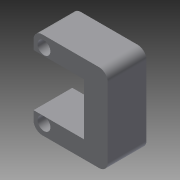
# Autodesk Inventor part: thermo-model
Saved by Autodesk Inventor 2014 (Build 180170000, 170)
## iProperties
Created: 2014-07-20
Part Number: thermo-model
Material: Generic
Document SubType Name: Modeling
Designer: james
Density: 1 g/cm^3
Appearance: Default
Author: james
Autodesk Inventor part; units mm, degrees
ref_plane "YZ Plane" through (0, 0, 0) normal (1, 0, 0) x (0, 1, 0)
ref_plane "XZ Plane" through (0, 0, 0) normal (0, 1, 0) x (-1, 0, 0)
ref_plane "XY Plane" through (0, 0, 0) normal (0, 0, 1) x (1, 0, 0)
sketch "Sketch1" plane through (0, 0, 0) normal (0, 1, 0) x (-1, 0, 0)
  spline S0 degree 3 poles (19.0088, -20.3781) (18.4587, -20.3781) (18.0142, -19.9334) (18.0142, -19.3832) (18.0142, -18.833) (18.4587, -18.3883) (19.0088, -18.3883) (19.5594, -18.3883) (20.0038, -18.833) (20.0038, -19.3832) (20.0038, -19.9334) (19.5594, -20.3781) (19.0088, -20.3781) knots 0 0 0 0 1 1 1 2 2 2 3 3 3 4 4 4 4
  line L0 (19.0088, -20.3781) -> (18.4587, -20.3781) construction
  line L1 (18.4587, -20.3781) -> (18.0142, -19.9334) construction
  line L2 (18.0142, -19.9334) -> (18.0142, -19.3832) construction
  line L3 (18.0142, -19.3832) -> (18.0142, -18.833) construction
  line L4 (18.0142, -18.833) -> (18.4587, -18.3883) construction
  line L5 (18.4587, -18.3883) -> (19.0088, -18.3883) construction
  line L6 (19.0088, -18.3883) -> (19.5594, -18.3883) construction
  line L7 (19.5594, -18.3883) -> (20.0038, -18.833) construction
  line L8 (20.0038, -18.833) -> (20.0038, -19.3832) construction
  line L9 (20.0038, -19.3832) -> (20.0038, -19.9334) construction
  line L10 (20.0038, -19.9334) -> (19.5594, -20.3781) construction
  line L11 (19.5594, -20.3781) -> (19.0088, -20.3781) construction
  spline S1 degree 3 poles (19.0088, -20.3781) (18.4587, -20.3781) (18.0142, -19.9334) (18.0142, -19.3832) (18.0142, -18.833) (18.4587, -18.3883) (19.0088, -18.3883) (19.5594, -18.3883) (20.0038, -18.833) (20.0038, -19.3832) (20.0038, -19.9334) (19.5594, -20.3781) (19.0088, -20.3781) knots 0 0 0 0 1 1 1 2 2 2 3 3 3 4 4 4 4
  line L12 (19.0088, -20.3781) -> (18.4587, -20.3781) construction
  line L13 (18.4587, -20.3781) -> (18.0142, -19.9334) construction
  line L14 (18.0142, -19.9334) -> (18.0142, -19.3832) construction
  line L15 (18.0142, -19.3832) -> (18.0142, -18.833) construction
  line L16 (18.0142, -18.833) -> (18.4587, -18.3883) construction
  line L17 (18.4587, -18.3883) -> (19.0088, -18.3883) construction
  line L18 (19.0088, -18.3883) -> (19.5594, -18.3883) construction
  line L19 (19.5594, -18.3883) -> (20.0038, -18.833) construction
  line L20 (20.0038, -18.833) -> (20.0038, -19.3832) construction
  line L21 (20.0038, -19.3832) -> (20.0038, -19.9334) construction
  line L22 (20.0038, -19.9334) -> (19.5594, -20.3781) construction
  line L23 (19.5594, -20.3781) -> (19.0088, -20.3781) construction
  spline S2 degree 3 poles (19.0088, -5.1804) (18.4587, -5.1804) (18.0142, -4.7359) (18.0142, -4.1855) (18.0142, -3.6352) (18.4587, -3.1907) (19.0088, -3.1907) (19.5594, -3.1907) (20.0038, -3.6352) (20.0038, -4.1855) (20.0038, -4.7359) (19.5594, -5.1804) (19.0088, -5.1804) knots 0 0 0 0 1 1 1 2 2 2 3 3 3 4 4 4 4
  line L24 (19.0088, -5.1804) -> (18.4587, -5.1804) construction
  line L25 (18.4587, -5.1804) -> (18.0142, -4.7359) construction
  line L26 (18.0142, -4.7359) -> (18.0142, -4.1855) construction
  line L27 (18.0142, -4.1855) -> (18.0142, -3.6352) construction
  line L28 (18.0142, -3.6352) -> (18.4587, -3.1907) construction
  line L29 (18.4587, -3.1907) -> (19.0088, -3.1907) construction
  line L30 (19.0088, -3.1907) -> (19.5594, -3.1907) construction
  line L31 (19.5594, -3.1907) -> (20.0038, -3.6352) construction
  line L32 (20.0038, -3.6352) -> (20.0038, -4.1855) construction
  line L33 (20.0038, -4.1855) -> (20.0038, -4.7359) construction
  line L34 (20.0038, -4.7359) -> (19.5594, -5.1804) construction
  line L35 (19.5594, -5.1804) -> (19.0088, -5.1804) construction
  spline S3 degree 3 poles (19.0088, -5.1804) (18.4587, -5.1804) (18.0142, -4.7359) (18.0142, -4.1855) (18.0142, -3.6352) (18.4587, -3.1907) (19.0088, -3.1907) (19.5594, -3.1907) (20.0038, -3.6352) (20.0038, -4.1855) (20.0038, -4.7359) (19.5594, -5.1804) (19.0088, -5.1804) knots 0 0 0 0 1 1 1 2 2 2 3 3 3 4 4 4 4
  line L36 (19.0088, -5.1804) -> (18.4587, -5.1804) construction
  line L37 (18.4587, -5.1804) -> (18.0142, -4.7359) construction
  line L38 (18.0142, -4.7359) -> (18.0142, -4.1855) construction
  line L39 (18.0142, -4.1855) -> (18.0142, -3.6352) construction
  line L40 (18.0142, -3.6352) -> (18.4587, -3.1907) construction
  line L41 (18.4587, -3.1907) -> (19.0088, -3.1907) construction
  line L42 (19.0088, -3.1907) -> (19.5594, -3.1907) construction
  line L43 (19.5594, -3.1907) -> (20.0038, -3.6352) construction
  line L44 (20.0038, -3.6352) -> (20.0038, -4.1855) construction
  line L45 (20.0038, -4.1855) -> (20.0038, -4.7359) construction
  line L46 (20.0038, -4.7359) -> (19.5594, -5.1804) construction
  line L47 (19.5594, -5.1804) -> (19.0088, -5.1804) construction
  line L48 (19.0302, -21.9233) -> (19.4746, -21.9019)
  spline S4 degree 3 poles (19.4746, -21.9019) (20.5647, -21.6366) (21.3157, -20.9538) (21.5279, -19.8276) knots 1 1 1 1 2 2 2 2
  line L49 (19.4746, -21.9019) -> (20.5647, -21.6366) construction
  line L50 (20.5647, -21.6366) -> (21.3157, -20.9538) construction
  line L51 (21.3157, -20.9538) -> (21.5279, -19.8276) construction
  line L52 (21.5279, -19.8276) -> (21.5703, -19.4042)
  line L53 (21.5703, -19.4042) -> (21.5703, -4.1855)
  line L54 (21.5703, -4.1855) -> (21.5279, -3.7411)
  spline S5 degree 3 poles (21.5279, -3.7411) (21.3143, -2.6778) (20.5474, -1.8728) (19.4746, -1.6878) knots 5 5 5 5 6 6 6 6
  line L55 (21.5279, -3.7411) -> (21.3143, -2.6778) construction
  line L56 (21.3143, -2.6778) -> (20.5474, -1.8728) construction
  line L57 (20.5474, -1.8728) -> (19.4746, -1.6878) construction
  line L58 (19.4746, -1.6878) -> (19.0302, -1.6456)
  line L59 (19.0302, -1.6456) -> (3.8115, -1.6456)
  line L60 (3.8115, -1.6456) -> (3.3881, -1.6878)
  spline S6 degree 3 poles (3.3881, -1.6878) (2.3177, -1.8298) (1.536, -2.7195) (1.3138, -3.7411) knots 9 9 9 9 10 10 10 10
  line L61 (3.3881, -1.6878) -> (2.3177, -1.8298) construction
  line L62 (2.3177, -1.8298) -> (1.536, -2.7195) construction
  line L63 (1.536, -2.7195) -> (1.3138, -3.7411) construction
  line L64 (1.3138, -3.7411) -> (1.2924, -4.1855)
  line L65 (1.2924, -4.1855) -> (1.2924, -19.4042)
  line L66 (1.2924, -19.4042) -> (1.3138, -19.8276)
  spline S7 degree 3 poles (1.3138, -19.8276) (1.5308, -20.908) (2.308, -21.6852) (3.3881, -21.9019) knots 13 13 13 13 14 14 14 14
  line L67 (1.3138, -19.8276) -> (1.5308, -20.908) construction
  line L68 (1.5308, -20.908) -> (2.308, -21.6852) construction
  line L69 (2.308, -21.6852) -> (3.3881, -21.9019) construction
  line L70 (3.3881, -21.9019) -> (3.8115, -21.9233)
  line L71 (3.8115, -21.9233) -> (19.0302, -21.9233)
  point P0 (0, 0)
  constraints: 24 end point, 20 other
sketch "Sketch2" plane through (0, 0, 0) normal (0, 1, 0) x (-1, 0, 0)
  line L0 (19.5198, -21.9426) -> (6.2891, -21.9426)
  line L1 (4.2891, -19.9426) -> (4.2891, -3.657)
  line L2 (6.2891, -1.657) -> (19.5198, -1.657)
  line L3 (21.5198, -3.657) -> (21.5198, -19.9426)
  arc A0 (21.5198, -3.657) -> (19.5198, -1.657) centre (19.5198, -3.657) ccw
  arc A1 (19.5198, -21.9426) -> (21.5198, -19.9426) centre (19.5198, -19.9426) ccw
  arc A2 (4.2891, -19.9426) -> (6.2891, -21.9426) centre (6.2891, -19.9426) ccw
  arc A3 (6.2891, -1.657) -> (4.2891, -3.657) centre (6.2891, -3.657) ccw
  circle A4 centre (19.1022, -4.1405) radius 1.5
  circle A5 centre (19.1022, -19.4152) radius 1.5
  line L4 (21.5198, -5.825) -> (9.7891, -5.825)
  line L5 (9.7891, -5.825) -> (9.7891, -17.9152)
  line L6 (9.7891, -17.9152) -> (21.5198, -17.9152)
  point P0 (0, 0)
  dimension "d0" = 2
  dimension "d1" = 3
  dimension "d2" = 3
  constraints: 14 end point, 8 point on circle, 8 tangent, 6 centre point, 3 equal radius, 3 perpendicular, 2 parallel, 2 point on line, 1 horizontal
  measures "d0" radius of A0
  measures "d1" diameter of A4
  measures "d2" diameter of A5
extrude "Extrusion1" add sketch "Sketch2" along normal blind 9 contours L0 A2 L1 A3 L2 A0 L3 L4 L5 L6 A1
body "Solid1"
